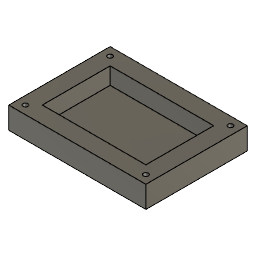
ArxHackapad (Assembly) (Autodesk Fusion 360 archive; units mm, degrees)
design "ArxHackapad"
part number: 2026-03-30-11-25-55-804
Autodesk Fusion 360 part; units mm, degrees
sketch "Sketch2" plane through (0, 0, 0) normal (0, 0, 1) x (1, 0, 0)
  line L0 (0, 0) -> (61.5, 0)
  line L1 (61.5, 0) -> (61.5, 40.25)
  line L2 (61.5, 40.25) -> (0, 40.25)
  line L3 (0, 40.25) -> (0, 0)
  line L4 (-10, 50.25) -> (71.5, 50.25)
  line L5 (71.5, 50.25) -> (71.5, -10)
  line L6 (71.5, -10) -> (-10, -10)
  line L7 (-10, -10) -> (-10, 50.25)
  circle A0 centre (-5, 45.25) radius 1.45
  circle A1 centre (-5, -5) radius 1.45
  circle A2 centre (66.5, 45.25) radius 1.45
  circle A3 centre (66.5, -5) radius 1.45
  dimension "d1" = 61.5
  dimension "d2" = 40.25
  dimension "d3" = 81.5
  dimension "d4" = 60.25
  dimension "d5" = 10
  dimension "d6" = 10
  dimension "d7" = 2.9
  dimension "d8" = 5
  dimension "d9" = 5
  dimension "d10" = 2.9
  dimension "d11" = 5
  dimension "d12" = 5
  dimension "d13" = 2.9
  dimension "d14" = 5
  dimension "d15" = 5
  dimension "d16" = 2.9
  dimension "d17" = 5
  dimension "d18" = 5
  constraint horizontal L0
  constraint vertical L1
  constraint horizontal L2
  constraint vertical L3
  constraint coincident L0.start L3.end
  constraint horizontal L4
  constraint vertical L5
  constraint horizontal L6
  constraint vertical L7
  measures "d1" distance of L0.start L0.end
  measures "d2" distance of L0.start L2.end
  measures "d3" distance of L4.start L4.end
  measures "d4" distance of L4.start L6.end
  measures "d5" distance of L2 L4
  measures "d6" distance of L3 L7
  measures "d7" diameter of A0
  measures "d8" distance of L4 A0.centre
  measures "d9" distance of L7 A0.centre
  measures "d10" diameter of A1
  measures "d11" distance of L6 A1.centre
  measures "d12" distance of L7 A1.centre
  measures "d13" diameter of A2
  measures "d14" distance of L4 A2.centre
  measures "d15" distance of L5 A2.centre
  measures "d16" diameter of A3
  measures "d17" distance of L5 A3.centre
  measures "d18" distance of L6 A3.centre
extrude "Extrude3" add sketch "Sketch2" along normal blind 13
extrude "Extrude4" add sketch "Sketch2" along normal blind 3 contours L0 L1 L2 L3
